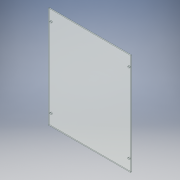
# Autodesk Inventor part: perspex height
Saved by Autodesk Inventor 2019 (Build 230136000, 136)
## iProperties
Created: 2021-03-22
Part Number: perspex height
Material: Glass
Document SubType Name: Modeling
Designer: User
Density: 2.18 g/cm^3
Appearance: Clear
Author: User
Autodesk Inventor part; units mm, degrees
ref_plane "YZ Plane" through (0, 0, 0) normal (1, 0, 0) x (0, 1, 0)
ref_plane "XZ Plane" through (0, 0, 0) normal (0, 1, 0) x (-1, 0, 0)
ref_plane "XY Plane" through (0, 0, 0) normal (0, 0, 1) x (1, 0, 0)
sketch "Sketch1" plane through (0, 0, 0) normal (0, 0, 1) x (1, 0, 0)
  line L0 (0, 0) -> (373, 0)
  line L1 (373, 0) -> (373, 460)
  line L2 (373, 460) -> (0, 460)
  line L3 (0, 460) -> (0, 0)
  dimension "d0" = 373
  dimension "d1" = 460
  constraints: 8 end point, 2 parallel, 1 horizontal, 1 perpendicular
  measures "d0" distance between parallel lines of L1 L3
  measures "d1" distance between parallel lines of L2 L0
extrude "Extrusion1" add sketch "Sketch1" along normal mid plane 4
sketch "Sketch2" plane through (0, 0, 2) normal (0, 0, 1) x (1, 0, 0)
  circle A0 centre (9.5, 410) radius 4
  circle A1 centre (363.5, 410) radius 4
  circle A2 centre (9.5, 50) radius 4
  circle A3 centre (363.5, 50) radius 4
  line L0 (373, 460) -> (0, 460) projected
  line L1 (373, 0) -> (373, 460) projected
  line L2 (0, 460) -> (0, 0) projected
  line L3 (0, 0) -> (373, 0) projected
  dimension "d4" = 8
  dimension "d5" = 8
  dimension "d6" = 8
  dimension "d7" = 8
  dimension "d8" = 50
  dimension "d9" = 9.5
  dimension "d10" = 50
  dimension "d11" = 9.5
  dimension "d12" = 50
  dimension "d13" = 9.5
  dimension "d14" = 50
  dimension "d15" = 9.5
  constraints: 4 centre point
  measures "d4" diameter of A0
  measures "d5" diameter of A1
  measures "d6" diameter of A2
  measures "d7" diameter of A3
  measures "d8" distance from line of A1.centre L0
  measures "d9" distance from line of L1 A1.centre
  measures "d10" distance from line of L0 A0.centre
  measures "d11" distance from line of L2 A0.centre
  measures "d12" distance from line of A2.centre L3
  measures "d13" distance from line of L2 A2.centre
  measures "d14" distance from line of L3 A3.centre
  measures "d15" distance from line of L1 A3.centre
extrude "Extrusion2" cut sketch "Sketch2" against normal blind 4 contours A0 | A1 | A2 | A3
body "Solid1"
